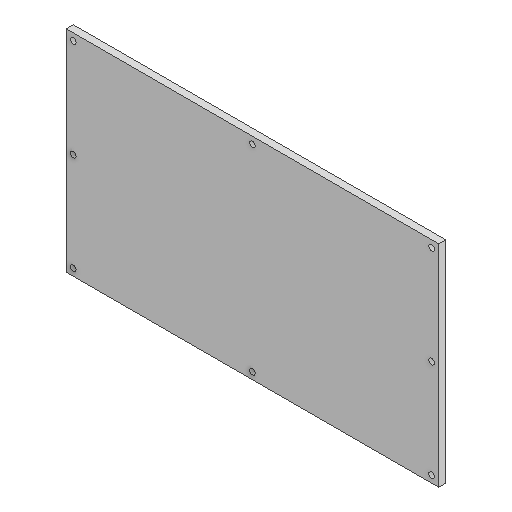
# Autodesk Inventor part: Tapa
Saved by Autodesk Inventor 2025.2 (Build 292293000, 293)
## iProperties
Created: 2025-08-05
Part Number: Tapa
Material: Generic
Document SubType Name: Modeling
Designer: Compa
Density: 1 g/cm^3
Appearance: Default
Author: Compa
Autodesk Inventor part; units mm, degrees
ref_plane "YZ Plane" through (0, 0, 0) normal (1, 0, 0) x (0, 1, 0)
ref_plane "XZ Plane" through (0, 0, 0) normal (0, 1, 0) x (-1, 0, 0)
ref_plane "XY Plane" through (0, 0, 0) normal (0, 0, 1) x (1, 0, 0)
sketch "Sketch1" plane through (0, 0, 0) normal (0, 0, 1) x (1, 0, 0)
  line L0 (0, 0) -> (265, 0)
  line L1 (0, 0) -> (0, -150)
  line L2 (0, -150) -> (265, -150)
  line L3 (265, -150) -> (265, 0)
  line L4 (260, -5) -> (5, -5)
  line L5 (5, -5) -> (5, -145)
  line L6 (5, -145) -> (260, -145)
  line L7 (260, -145) -> (260, -5)
  circle A0 centre (5, -5) radius 5
  circle A1 centre (5, -5) radius 2.05
  circle A2 centre (260, -5) radius 5
  circle A3 centre (260, -5) radius 2.05
  circle A4 centre (5, -145) radius 5
  circle A5 centre (5, -145) radius 2.05
  circle A6 centre (260, -145) radius 5
  circle A7 centre (260, -145) radius 2.05
  line L8 (5, -5) -> (5, -75)
  circle A8 centre (5, -75) radius 5
  circle A9 centre (5, -75) radius 2.05
  line L9 (260, -5) -> (260, -75)
  circle A10 centre (260, -75) radius 5
  circle A11 centre (260, -75) radius 2.05
  line L10 (5, -5) -> (132.5, -5)
  circle A12 centre (132.5, -5) radius 5
  circle A13 centre (132.5, -5) radius 2.05
  line L11 (5, -145) -> (132.5, -145)
  circle A14 centre (132.5, -145) radius 5
  circle A15 centre (132.5, -145) radius 2.05
  dimension "d0" = 265
  dimension "d1" = 150
  dimension "d2" = 265
  dimension "d3" = 5
  dimension "d4" = 10
  dimension "d5" = 4.1
  dimension "d6" = 10
  dimension "d7" = 4.1
  dimension "d8" = 10
  dimension "d9" = 4.1
  dimension "d10" = 10
  dimension "d11" = 4.1
  dimension "d12" = 70
  dimension "d13" = 10
  dimension "d14" = 4.1
  dimension "d15" = 70
  dimension "d16" = 10
  dimension "d17" = 4.1
  dimension "d18" = 127.5
  dimension "d19" = 10
  dimension "d20" = 4.1
  dimension "d21" = 127.5
  dimension "d22" = 10
  dimension "d23" = 4.1
  constraints: 24 end point, 16 centre point, 16 coincident, 4 midpoint, 2 perpendicular, 1 horizontal, 1 vertical, 3 other
  measures "d0" distance of L0.start L0.end
  measures "d1" distance of L0.start L1.end
  measures "d2" distance of L1.end L2.end
  measures "d3" distance between parallel lines of L0 L4
  measures "d4" diameter of A0
  measures "d5" diameter of A1
  measures "d6" diameter of A2
  measures "d7" diameter of A3
  measures "d8" diameter of A4
  measures "d9" diameter of A5
  measures "d10" diameter of A6
  measures "d11" diameter of A7
  measures "d12" distance of L8.start L8.end
  measures "d13" diameter of A8
  measures "d14" diameter of A9
  measures "d15" distance of L9.start L9.end
  measures "d16" diameter of A10
  measures "d17" diameter of A11
  measures "d18" distance of L8.start L10.end
  measures "d19" diameter of A12
  measures "d20" diameter of A13
  measures "d21" distance of L11.start L11.end
  measures "d22" diameter of A14
  measures "d23" diameter of A15
extrude "Extrusion1" add sketch "Sketch1" along normal blind 5 contours L0 A0 L1 | L0 A12 L4 A0 | A0 L4 A1 L5 | A0 L5 A8 L1 | L0 A2 L4 A12 | A12 L4 A13 | A0 L5 A1 L4 | L4 A12 A2 L7 A10 A6 L6 A14 A4 L5 A8 A0 | A8 L5 A4 L1 | A8 L5 A9 | L0 L3 A2 | A2 L7 A3 L4 | A12 L4 A13 | A4 L2 L1 | A4 L5 A5 L6 | A8 L5 A9 | L3 A10 L7 A2 | L4 A3 L7 A2 | A4 L6 A5 L5 | A4 L6 A14 L2 | A10 L7 A11 | L3 A6 L7 A10 | A14 L6 A6 L2 | A14 L6 A15 | A6 L6 A7 L7 | L3 L2 A6 | L7 A11 A10 | A14 L6 A15 | L7 A7 L6 A6
body "Solid1"
